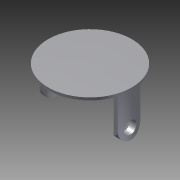
# Autodesk Inventor part: SB4011NO-trmnls
Saved by Autodesk Inventor 2014 (Build 180170000, 170)
## iProperties
Category: PARTsolutions
Company: NKKSWITCHES
Created: 2013-12-28
Part Number: SB4011NO-trmnls
Catalog Web Link: www.cadenas.de
Description: SB4011 Series - 3 Amp Momentary Pushbuttons -trmnls-
Vendor: NKKSWITCHES
Document SubType Name: Modeling
Designer: PARTuser1
Manufacturer: NKKSWITCHES
Density: 1 g/cm^3
Material: Generic
Appearance: RGB(191.25000000000000,191.25000000000000,191.25000000000000)
PSOL_IDENT_0: {$CADENAS_DATA\23d-libs\nkkswitches\pushbuttons\sb4011\parts\sb4011_trmnls.prj},229 {VTYP=3D},{NB=SB
PSOL_IDENT_1: 4011NO-trmnls},{LINA=SB4011NO-trmnls},{NN=SB4011 Series - 3 Amp Momentary Pushbuttons -trmnls},{DATE
PSOL_IDENT_2: =17.02.2009 10:23:06},{GEOMDATE=16.02.2009 06:33:00},{VERSION=},{LINEID=10},{LINESUBID=-1},{WBVAR=PL
PSOL_IDENT_3: SCRCTS,CMR}  {NB=SB4011NO-trmnls},{LINA=SB4011NO-trmnls},{KT=DUMMY},{PN=SB4011NO},{SRS=SB40},{PLSCRC
PSOL_IDENT_4: TS=11NO},{CMR=},{CMRALG= 0.75,0.75,0.75,0.00 },{TL=0.157}
CNS_NN: SB4011 Series - 3 Amp Momentary Pushbuttons -trmnls
CNS_NB: SB4011NO-trmnls
CNS_NBSYN: $PN.-trmnls
CNS_LINA: SB4011NO-trmnls
CNS_PN: SB4011NO
CNS_SRS: SB40
CNS_PLSCRCTS: 11NO - SPST/OFF/(ON) (Normally Open)
CNS_CMR: Silver Contacts 3A @ 125V AC or 2A @ 250V DC
CNS_CMRALG: 0.75,0.75,0.75,0.00
CNS_TL: 0.157
SUPPLIER: NKKSWITCHES
ARTICLENO: SB4011NO-trmnls
BOMINFO: SB4011NO-trmnls
CREATOR: CADENAS GmbH
Title: SB4011NO-trmnls
Author: Cadenas PARTsolutions
Autodesk Inventor part; units mm, degrees
sketch "Sketch_2" plane through (0, 0, 0) normal (0, 1, 0) x (-1, 0, 0)
  circle A0 centre (0, 0) radius 4.064
  constraints: 1 centre point
extrude "Extrusion1" add sketch "Sketch_2" along normal blind 0.254
sketch "Sketch_3" plane through (0, 0, 0) normal (0, 1, 0) x (-1, 0, 0)
  arc A0 (-3.2099, 0.9236) -> (-3.2099, -0.9236) centre (0, 0) ccw
  line L0 (-3.2099, 0.9236) -> (-3.7957, 1.0922)
  arc A1 (-3.7957, 1.0922) -> (-3.7957, -1.0922) centre (0, 0) ccw
  line L1 (-3.7957, -1.0922) -> (-3.2099, -0.9236)
  constraints: 4 end point, 4 point on circle, 2 centre point
extrude "Extrusion2" add sketch "Sketch_3" against normal blind 4.2418
sketch "Sketch_4" plane through (0, 0, 0) normal (0, 1, 0) x (-1, 0, 0)
  arc A0 (3.7957, -1.0922) -> (3.7957, 1.0922) centre (0, 0) ccw
  line L0 (3.7957, 1.0922) -> (3.2099, 0.9236)
  arc A1 (3.2099, -0.9236) -> (3.2099, 0.9236) centre (0, 0) ccw
  line L1 (3.2099, -0.9236) -> (3.7957, -1.0922)
  constraints: 4 end point, 4 point on circle, 2 centre point
extrude "Extrusion3" add sketch "Sketch_4" against normal blind 4.2418
sketch "Sketch_5" plane through (0, 0, 0) normal (1, 0, 0) x (0, 1, 0)
  circle A0 centre (-3.175, 0) radius 0.5969
  constraints: 1 centre point
extrude "Extrusion4" cut sketch "Sketch_5" along normal mid plane 16.3576
sketch "Sketch_6" plane through (0, 0, 0) normal (1, 0, 0) x (0, 1, 0)
  line L0 (-4.4958, 1.0922) -> (-4.4958, -1.0922)
  line L1 (-4.4958, -1.0922) -> (-3.175, -1.0922)
  arc A0 (-3.175, 1.0922) -> (-3.175, -1.0922) centre (-3.1493, 0) ccw
  line L2 (-3.175, 1.0922) -> (-4.4958, 1.0922)
  constraints: 6 end point, 2 point on circle, 1 centre point
extrude "Extrusion5" cut sketch "Sketch_6" along normal mid plane 16.3576
ref_plane "to_trmnl_hold_XY" through (0, 0, 0) normal (0, -1, 0) x (1, 0, 0)
ref_plane "to_trmnl_hold_YZ" through (0, 0, 0) normal (1, 0, 0) x (0, 0, 1)
ref_plane "to_trmnl_hold_ZX" through (0, 0, 0) normal (0, 0, 1) x (0, -1, 0)
body "Solid1"
